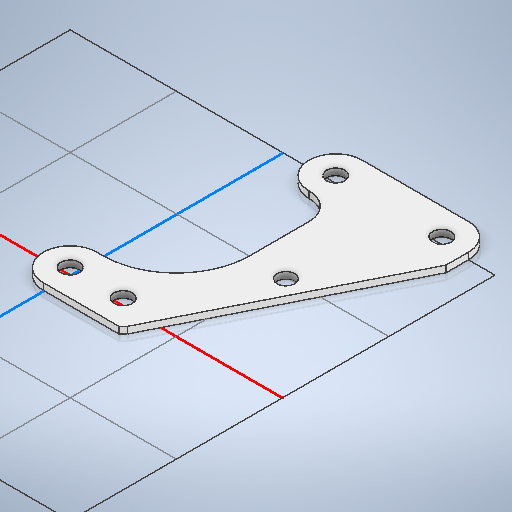
# Autodesk Inventor part: Front Gusset
Saved by Autodesk Inventor 2026 (Build 300175000, 175)
## iProperties
Created: 2025-04-05
Part Number: Front Gusset
Material: Acetal Resin, White
Document SubType Name: Modeling
Designer: avere
Density: 1.425 g/cm^3
Appearance: Smooth - White
Author: avere
Autodesk Inventor part; units mm, degrees
ref_plane "YZ Plane" through (0, 0, 0) normal (1, 0, 0) x (0, 1, 0)
ref_plane "XZ Plane" through (0, 0, 0) normal (0, 1, 0) x (-1, 0, 0)
ref_plane "XY Plane" through (0, 0, 0) normal (0, 0, 1) x (1, 0, 0)
sketch "main" plane through (0, 0, 0) normal (0, 0, 1) x (1, 0, 0)
  circle A0 centre (11.2296, 26.3602) radius 2.1844
  line L0 (23.9296, 20.0102) -> (22.6596, 20.0102)
  line L1 (4.8796, 31.6942) -> (5.8956, 32.7102)
  circle A1 centre (23.9296, 26.3602) radius 2.1844
  line L2 (23.9296, 32.7102) -> (5.8956, 32.7102)
  arc A2 (23.9296, 20.0102) -> (23.9296, 32.7102) centre (23.9296, 26.3602) ccw
  circle A3 centre (-14.1704, -24.4398) radius 2.1844
  circle A4 centre (11.2296, -24.4398) radius 2.1844
  arc A5 (22.6596, 20.0102) -> (4.8796, 2.2302) centre (22.6596, 2.2302) ccw
  line L3 (4.8796, -11.7398) -> (4.8796, 2.2302)
  arc A6 (4.8796, -11.7398) -> (11.2296, -18.0898) centre (11.2296, -11.7398) ccw
  line L4 (4.8796, 31.6942) -> (-20.5204, -19.1058)
  arc A7 (11.2296, -30.7898) -> (11.2296, -18.0898) centre (11.2296, -24.4398) ccw
  line L5 (11.2296, -30.7898) -> (-14.1704, -30.7898)
  line L6 (-20.5204, -24.4398) -> (-20.5204, -19.1058)
  arc A8 (-20.5204, -24.4398) -> (-14.1704, -30.7898) centre (-14.1704, -24.4398) ccw
  circle A9 centre (-4.1968, 2.8922) radius 2.0955
  point P0 (6.0044, -0.2269)
  dimension "d0" = 12.7
  dimension "d1" = 17.78
  dimension "d2" = 6.35
  dimension "d3" = 1.27
  dimension "d4" = 6.35
  dimension "d8" = 4.191
  measures "d0" diameter of A8
  measures "d1" radius of A5
  measures "d2" radius of A6
  measures "d3" distance of L0.start L0.end
  measures "d4" radius of A7
  measures "d8" diameter of A9
sketch "Sketch1" plane through (0, 0, 0) normal (0, 1, 0) x (-1, 0, 0)
  circle A0 centre (-12.7, 0) radius 2.1844
  line L0 (0, -6.35) -> (-1.27, -6.35)
  line L1 (-19.05, 5.334) -> (-18.034, 6.35)
  circle A1 centre (0, 0) radius 2.1844
  line L2 (0, 6.35) -> (-18.034, 6.35)
  arc A2 (0, -6.35) -> (0, 6.35) centre (0, 0) ccw
  circle A3 centre (-38.1, -50.8) radius 2.1844
  circle A4 centre (-12.7, -50.8) radius 2.1844
  arc A5 (-1.27, -6.35) -> (-19.05, -24.13) centre (-1.27, -24.13) ccw
  line L3 (-19.05, -38.1) -> (-19.05, -24.13)
  arc A6 (-19.05, -38.1) -> (-12.7, -44.45) centre (-12.7, -38.1) ccw
  line L4 (-19.05, 5.334) -> (-44.45, -45.466)
  arc A7 (-12.7, -57.15) -> (-12.7, -44.45) centre (-12.7, -50.8) ccw
  line L5 (-12.7, -57.15) -> (-38.1, -57.15)
  line L6 (-44.45, -50.8) -> (-44.45, -45.466)
  arc A8 (-44.45, -50.8) -> (-38.1, -57.15) centre (-38.1, -50.8) ccw
  circle A9 centre (-28.1264, -23.468) radius 2.0955
  constraints: 1 other
extrude "Extrusion1" add sketch "Sketch1" along normal blind 1.5875
body "Solid1"
